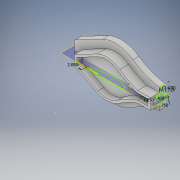
# Autodesk Inventor part: thingymajig
Saved by Autodesk Inventor 2018 (Build 220112000, 112)
## iProperties
Created: 2018-03-12
Part Number: thingymajig
Material: Generic
Document SubType Name: Modeling
Designer: 232963
Density: 1 g/cm^3
Appearance: Default
Author: 232963
Autodesk Inventor part; units mm, degrees
ref_plane "YZ Plane" through (0, 0, 0) normal (1, 0, 0) x (0, 1, 0)
ref_plane "XZ Plane" through (0, 0, 0) normal (0, 1, 0) x (-1, 0, 0)
ref_plane "XY Plane" through (0, 0, 0) normal (0, 0, 1) x (1, 0, 0)
sketch "Sketch1" plane through (0, 0, 0) normal (0, 0, 1) x (1, 0, 0)
  line L0 (106.83, 41.275) -> (112.0189, 41.275)
  line L1 (180.975, 43.6569) -> (180.975, -43.6569)
  line L2 (-180.975, -34.2283) -> (-180.975, 34.2283)
  line L3 (-177.5333, 39.8732) -> (-61.7664, 99.5173)
  ellipse E0 centre (0, 0) end of major axis (-42.3691, -102.7308) minor radius 120.65 (68.3103, 88.3967) -> (-61.7664, 99.5173) ccw
  arc A0 (68.3103, 88.3967) -> (180.975, 43.6569) centre (215.6784, 295.275) ccw
  line L4 (-180.975, 0) -> (180.975, 0)
  line L5 (180.975, -43.6569) -> (180.975, 43.6569)
  line L6 (-180.975, 34.2283) -> (-180.975, -34.2283)
  line L7 (-177.5333, -39.8732) -> (-61.7664, -99.5173)
  ellipse E1 centre (0, 0) end of major axis (-42.3691, 102.7308) minor radius 120.65 (-61.7664, -99.5173) -> (68.3103, -88.3967) ccw
  arc A1 (180.975, -43.6569) -> (68.3103, -88.3967) centre (215.6784, -295.275) ccw
  arc A2 (-177.5333, 39.8732) -> (-180.975, 34.2283) centre (-174.625, 34.2283) ccw
  arc A3 (-180.975, -34.2283) -> (-177.5333, -39.8732) centre (-174.625, -34.2283) ccw
  point P0 (-180.975, 38.1)
  point P1 (-180.975, -38.1)
  dimension "d9" = 111.125
  dimension "d12" = 120.65
  dimension "d5" = 180.975
  dimension "d6" = 41.275
  dimension "d13" = 254
  dimension "d14" = 361.95
  dimension "d15" = 6.35
  constraints: 16 end point, 8 point on circle, 7 symmetric about line, 5 tangent, 4 centre point, 4 point on line, 2 horizontal, 2 midpoint, 1 coincident, 1 equal radius, 1 parallel, 1 perpendicular, 11 other
  measures "d5" distance from line of L1 point (0, 0)
  measures "d6" distance from line of L0 point (0, 0)
  measures "d13" radius of A1
  measures "d14" distance of L4.end L4.start
  measures "d15" radius of A2
extrude "Extrusion1" add sketch "Sketch1" along normal blind 25.4 contours L1 L4 L2 A2 L3 E0 A0
mirror "Mirror1" about plane through (-180.975, 0, 0) normal (0, -1, 0) of "Extrusion1"
sketch "Sketch3" plane through (0, 0, 25.4) normal (0, 0, 1) x (1, 0, 0)
  line L0 (180.975, 43.6569) -> (180.975, -43.6569)
  line L1 (-180.975, -34.2283) -> (-180.975, 34.2283)
  line L2 (-177.5333, 39.8732) -> (-61.7664, 99.5173)
  ellipse E0 centre (0, 0) end of major axis (-42.3691, -102.7308) minor radius 120.65 (68.3103, 88.3967) -> (-61.7664, 99.5173) ccw
  arc A0 (68.3103, 88.3967) -> (180.975, 43.6569) centre (215.6784, 295.275) ccw
  line L3 (-180.975, 34.2283) -> (-180.975, -34.2283)
  line L4 (-177.5333, -39.8732) -> (-61.7664, -99.5173)
  ellipse E1 centre (0, 0) end of major axis (-42.3691, 102.7308) minor radius 120.65 (-61.7664, -99.5173) -> (68.3103, -88.3967) ccw
  arc A1 (180.975, -43.6569) -> (68.3103, -88.3967) centre (215.6784, -295.275) ccw
  line L5 (180.975, -43.6569) -> (180.975, 43.6569)
  arc A2 (-177.5333, 39.8732) -> (-180.975, 34.2283) centre (-174.625, 34.2283) ccw
  arc A3 (-180.975, -34.2283) -> (-177.5333, -39.8732) centre (-174.625, -34.2283) ccw
  line L6 (-143.0231, -21.937) -> (-143.0746, 21.9105)
  line L7 (-143.0746, 21.9105) -> (-47.225, 71.293)
  arc A4 (49.8893, 62.5369) -> (127.0049, 23.6317) centre (215.6784, 295.275) ccw
  arc A5 (127.847, -23.3583) -> (49.8893, -62.5369) centre (215.6784, -295.275) ccw
  line L8 (-47.225, -71.293) -> (-143.1355, -21.8791)
  line L9 (180.975, 43.6569) -> (180.975, -43.6569) projected
  line L10 (180.975, 23.6317) -> (127.0049, 23.6317)
  line L11 (127.847, -23.3583) -> (180.975, -23.3583)
  line L12 (180.975, -23.3583) -> (180.975, 23.6317)
  line L13 (-180.975, 0) -> (-143.0489, 0)
  spline S0 degree 5 poles (-47.225, 71.293) (-42.289, 73.8361) (-37.1355, 75.9573) (-31.821, 77.6477) (-17.6326, 80.9504) (-3.0018, 81.3685) (6.0134, 80.5554) (20.7306, 77.5049) (34.5698, 71.7794) (39.9128, 69.0839) (45.0333, 65.9961) (49.8893, 62.5369) knots 0 0 0 0 0 0 0.271031 0.271031 0.271031 0.708985 0.708985 0.708985 1 1 1 1 1 1
  spline S1 degree 5 poles (49.8893, -62.5369) (45.0333, -65.9961) (39.9128, -69.0839) (34.5698, -71.7794) (20.7306, -77.5049) (6.0134, -80.5554) (-3.0018, -81.3685) (-17.6326, -80.9504) (-31.821, -77.6477) (-37.1355, -75.9573) (-42.289, -73.8361) (-47.225, -71.293) knots 0 0 0 0 0 0 0.291015 0.291015 0.291015 0.728969 0.728969 0.728969 1 1 1 1 1 1
  point P0 (-180.975, 38.1)
  point P1 (-180.975, -38.1)
  dimension "d20" = 111.125
  dimension "d21" = 120.65
  dimension "d27" = 31.75
  dimension "d28" = 31.75
  dimension "d18" = 180.975
  dimension "d22" = 254
  dimension "d24" = 6.35
  constraints: 26 end point, 12 point on circle, 7 point on line, 6 centre point, 4 parallel, 4 tangent, 1 coincident, 1 equal radius, 1 horizontal, 1 midpoint, 16 other
  measures "d18" distance from line of L0 point (0, 0)
  measures "d22" radius of A1
  measures "d24" radius of A2
extrude "Extrusion2" add sketch "Sketch3" along normal blind 38.1 contours L0 L11 A5 S1 L8 L6 L7 S0 A4 L10
sketch "Sketch4" plane through (0, 0, 63.5) normal (0, 0, 1) x (1, 0, 0)
  ellipse E0 centre (0, 0) end of major axis (-42.3691, -102.7308) minor radius 120.65 (68.3103, 88.3967) -> (-61.7664, 99.5173) ccw
  ellipse E1 centre (0, 0) end of major axis (-42.3691, 102.7308) minor radius 120.65 (-61.7664, -99.5173) -> (68.3103, -88.3967) ccw
  arc A0 (68.3103, 88.3967) -> (180.975, 43.6569) centre (215.6784, 295.275) ccw
  arc A1 (180.975, -43.6569) -> (68.3103, -88.3967) centre (215.6784, -295.275) ccw
  line L0 (180.975, 43.6569) -> (180.975, -43.6569)
  line L1 (180.975, -43.6569) -> (180.975, 43.6569)
  line L2 (-177.5333, -39.8732) -> (-61.7664, -99.5173)
  arc A2 (-180.975, -34.2283) -> (-177.5333, -39.8732) centre (-174.625, -34.2283) ccw
  line L3 (-180.975, -34.2283) -> (-180.975, 34.2283)
  arc A3 (-177.5333, 39.8732) -> (-180.975, 34.2283) centre (-174.625, 34.2283) ccw
  line L4 (-177.5333, 39.8732) -> (-61.7664, 99.5173)
  line L5 (-180.975, 34.2283) -> (-180.975, -34.2283)
  line L6 (-143.0231, -21.937) -> (-143.0746, 21.9105)
  line L7 (-143.0746, 21.9105) -> (-47.225, 71.293)
  arc A4 (49.8893, 62.5369) -> (127.0049, 23.6317) centre (215.6784, 295.275) ccw
  arc A5 (127.847, -23.3583) -> (49.8893, -62.5369) centre (215.6784, -295.275) ccw
  line L8 (-47.225, -71.293) -> (-143.1355, -21.8791)
  line L9 (180.975, 43.6569) -> (180.975, -43.6569)
  line L10 (180.975, 23.6317) -> (127.0049, 23.6317)
  line L11 (127.847, -23.3583) -> (180.975, -23.3583)
  line L12 (180.975, -23.3583) -> (180.975, 23.6317)
  line L13 (-180.975, 0) -> (-143.0489, 0)
  line L14 (-42.8545, 62.8102) -> (-133.5252, 16.0958)
  line L15 (-133.5252, 16.0958) -> (-133.4869, -16.4966)
  line L16 (-43.0097, -63.1113) -> (-133.4869, -16.4966)
  arc A6 (126.2242, -12.9595) -> (43.856, -54.0673) centre (215.6784, -295.275) ccw
  line L17 (126.2242, -12.9595) -> (170.5762, -12.9595)
  line L18 (170.5762, -12.9595) -> (170.5762, 13.2329)
  line L19 (170.5762, 13.2329) -> (125.3658, 13.2329)
  arc A7 (43.856, 54.0673) -> (125.3658, 13.2329) centre (215.6784, 295.275) ccw
  arc A8 (43.856, 54.0673) -> (-42.8545, 62.8102) centre (-6.5084, -11.0769) ccw
  arc A9 (-43.0097, -63.1113) -> (43.856, -54.0673) centre (-6.2601, 5.602) ccw
  spline S0 degree 5 poles (-47.225, 71.293) (-42.289, 73.8361) (-37.1355, 75.9573) (-31.821, 77.6477) (-17.6326, 80.9504) (-3.0018, 81.3685) (6.0134, 80.5554) (20.7306, 77.5049) (34.5698, 71.7794) (39.9128, 69.0839) (45.0333, 65.9961) (49.8893, 62.5369) knots 0 0 0 0 0 0 0.271031 0.271031 0.271031 0.708985 0.708985 0.708985 1 1 1 1 1 1
  spline S1 degree 5 poles (49.8893, -62.5369) (45.0333, -65.9961) (39.9128, -69.0839) (34.5698, -71.7794) (20.7306, -77.5049) (6.0134, -80.5554) (-3.0018, -81.3685) (-17.6326, -80.9504) (-31.821, -77.6477) (-37.1355, -75.9573) (-42.289, -73.8361) (-47.225, -71.293) knots 0 0 0 0 0 0 0.291015 0.291015 0.291015 0.728969 0.728969 0.728969 1 1 1 1 1 1
  point P0 (0, 0)
  point P1 (-180.975, -38.1)
  point P2 (-180.975, 38.1)
  dimension "d35" = 111.125
  dimension "d36" = 120.65
  dimension "d39" = 31.75
  dimension "d40" = 31.75
  dimension "d34" = 180.975
  dimension "d37" = 254
  dimension "d38" = 6.35
  constraints: 40 end point, 21 point on circle, 10 centre point, 7 point on line, 6 parallel, 4 tangent, 1 coincident, 1 equal radius, 1 horizontal, 1 midpoint, 20 other
  measures "d34" distance from line of L0 point (0, 0)
  measures "d37" radius of A1
  measures "d38" radius of A3
extrude "Extrusion3" cut sketch "Sketch4" against normal blind 25.4 contours A8 A7 L19 L18 L17 A6 A9 L16 L15 L14
sketch "Sketch5" plane through (180.975, 43.6569, 25.4) normal (1, 0, 0) x (0, 0, -1)
  point P0 (25.4, -43.6569)
sketch "Sketch6" plane through (180.975, 43.6569, 25.4) normal (1, 0, 0) x (0, 0, -1)
  circle A0 centre (6.35, -43.6569) radius 23.495
  line L0 (25.4, 0) -> (25.4, -87.3138) projected
  line L1 (25.4, 0) -> (0, 0) projected
  point P0 (25.4, -43.6569)
  dimension "d44" = 19.05
  dimension "d45" = 46.99
  dimension "d46" = 87.3138
  dimension "d47" = 43.6569
  constraints: 1 centre point
  measures "d44" distance from line of L0 A0.centre
  measures "d45" diameter of A0
  measures "d46" distance of L0.start L0.end
  measures "d47" distance from line of L1 A0.centre
extrude "Extrusion4" add sketch "Sketch6" against normal blind 116.84
sketch "Sketch7" plane through (180.975, 43.6569, 25.4) normal (1, 0, 0) x (0, 0, -1)
  circle A0 centre (6.35, -43.6569) radius 23.495
  line L0 (25.4, 0) -> (25.4, -87.3138)
  line L1 (25.4, 0) -> (0, 0)
  circle A1 centre (6.35, -43.6569) radius 17.78
  point P0 (25.4, -43.6569)
  point P1 (25.4, -43.6569)
  dimension "d50" = 19.05
  dimension "d51" = 46.99
  dimension "d52" = 87.3138
  dimension "d53" = 43.6569
  dimension "d54" = 35.56
  constraints: 4 end point, 2 centre point, 1 coincident
  measures "d50" distance from line of L0 A0.centre
  measures "d51" diameter of A0
  measures "d52" distance of L0.start L0.end
  measures "d53" distance from line of L1 A0.centre
  measures "d54" diameter of A1
ref_plane "Work Plane1" through (125.3658, 0.1367, 63.5) normal (0, -1, 0) x (1, 0, 0)
sketch "Sketch8" plane through (125.3658, 0.1367, 63.5) normal (0, -1, 0) x (1, 0, 0)
  line L0 (-258.891, 0) -> (-168.2203, 0) projected
  line L1 (-268.3889, -38.1) -> (-268.3889, 0) projected
  arc A0 (-217.5889, 0) -> (-84.1786, -19.05) centre (-115.9924, 234.8246) ccw
  arc A1 (-61.2308, -10.5358) -> (-84.1786, -19.05) centre (-62.2353, -43.0105) ccw
  line L2 (-61.2308, 7.7441) -> (-215.9432, 5.6923)
  line L3 (-215.9432, 5.6923) -> (-217.5889, 0)
  line L4 (-61.2308, -10.5358) -> (-61.2308, 7.7441)
  line L5 (45.2104, -20.955) -> (-61.2308, -20.955) projected
  point P0 (-125.3658, -63.5)
  dimension "d55" = 50.8
  constraints: 6 end point, 4 point on circle, 2 centre point, 1 perpendicular, 1 point on line
  measures "d55" distance from line of L1 L3.end
equation "\"d5\" = 0.5 * d3"
equation "\"d6\" = 0.5 * d4"
equation "\"d18\" = 0.5 * d25"
equation "\"d34\" = 0.5 * d41"
equation "\"d47\" = 0.5 * d46"
equation "\"d53\" = 0.5 * d52"
equation "\"d3\" = 361.95"
equation "\"d4\" = 82.55"
equation "\"d25\" = 361.95"
equation "\"d41\" = 361.95"
body "Solid1"
